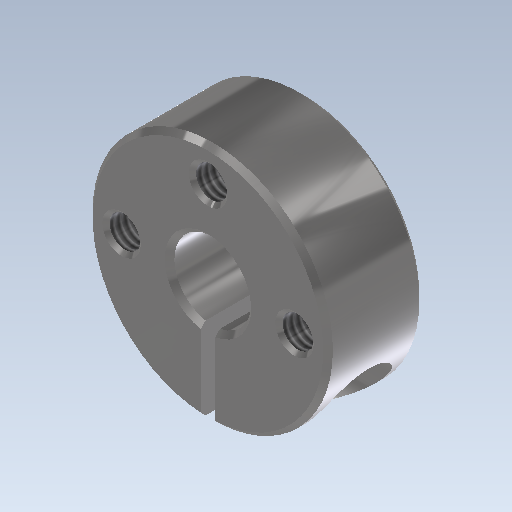
# Autodesk Inventor part: SCSTR8-10b
Saved by Autodesk Inventor 2020 (Build 240168000, 168)
## iProperties
Created: 2019-10-10
Part Number: SCSTR8-10b
Material: 鋼、炭素鋼
Catalog Web Link: www.cadenas.de
Description: SCST, PSCST, SSCST, SCSTR, PSCSTR, SSCSTR-b-Shaft Collars - 3 Holes/3 Taps
Vendor: MISUMI
Document SubType Name: Modeling
Designer: psadmin
Manufacturer: MISUMI
Mass: 28.8211 g
Surface Area: 23.8751 cm^2
Volume: 3.67148 cm^3
Density: 7.85 g/cm^3
Appearance: 半つや出し
Category: PARTsolutions
Company: MISUMI
PSOL_IDENT_0: {$CADENAS_DATA\23d-libs\misumi\metric\03_set_collars\scst\scst_b.prj},210 {VTYP=3D},{NB=SCSTR8-10b},
PSOL_IDENT_1: {LINA=SCSTR8-10},{NN=SCST, PSCST, SSCST, SCSTR, PSCSTR, SSCSTR-b},{DATE=30.03.2018 01:14:48},{GEOMDA
PSOL_IDENT_2: TE=30.10.2015 01:43:51},{VERSION=},{LINEID=50},{WBVAR=TS,MAT,ST,BS},{WBNUMERIC=BS}  {NB=SCSTR8-10b},
PSOL_IDENT_3: {LINA=SCSTR8-10},{KT=DUMMY},{PN=SCSTR8-10},{TYPE=SCSTR},{TS=3T},{TSALG= '3H' , '3-Hole' , '3T' , '3-
PSOL_IDENT_4: Tapped' },{TSA='3H', '3-Hole', '3T', '3 Tap (Coarse)'},{MAT=S45C},{ST=BO},{STALG= 'BO' , 'Black Oxid
PSOL_IDENT_5: e' , 'ENP' , 'Electroless Nickel Plating' },{AC=Hex Socket Head Cap Screw 1 pc.},{ACMAT=4137 Alloy S
PSOL_IDENT_6: teel},{D=8},{BS=10},{BALG= 8 , 10 },{D1=25},{M=M4},{M3D=4},{DD=4.5},{R=3.75},{W=1.5},{X=8.0},{Y=5},{
PSOL_IDENT_7: P=18},{C=0.5},{S=0.0},{M1=M4},{M13D=4},{L=12}
NN: SCST, PSCST, SSCST, SCSTR, PSCSTR, SSCSTR-b
NT: Shaft Collars - 3 Holes/3 Taps
NB: SCSTR8-10b
NBSYN: $PN.b
LINA: SCSTR8-10
PN: SCSTR8-10
TS: 3-Tapped
MAT: 1045 Carbon Steel
ST: Black Oxide
AC: Hex Socket Head Cap Screw 1 pc.
ACMAT: 4137 Alloy Steel
D: 8
BS: 10
D1: 25
M: M4
DD: 4.5
R: 3.75
W: 1.5
X: 8
Y: 5
P: 18
C: 0.5
S: 0
M1: M4
SUPPLIER: MISUMI
ARTICLENO: SCSTR8-10b
BOMINFO: SCSTR8-10
CREATOR: CADENAS GmbH
Title: SCSTR8-10
Author: Cadenas PARTsolutions
Comments: Shaft Collars - 3 Holes/3 Taps
Autodesk Inventor part; units mm, degrees
sketch "Sketch_14" plane through (0, 0, 0) normal (1, 0, 0) x (0, 1, 0)
  line L0 (0, -5) -> (0, 5)
  line L1 (0, 5) -> (12, 5)
  line L2 (12, 5) -> (12.5, 4.5)
  line L3 (12.5, 4.5) -> (12.5, -4.5)
  line L4 (12.5, -4.5) -> (12, -5)
  line L5 (12, -5) -> (0, -5)
  line L6 (0, -5) -> (0, 5)
  constraints: 14 end point
revolve "Revolution1" add sketch "Sketch_14" angle 360 about axis through (0, 0, -5) along (0, 0, -1)
sketch "Sketch_15" plane through (0, 0, 0) normal (1, 0, 0) x (0, 1, 0)
  line L0 (0, -5) -> (0, 5)
  line L1 (0, 5) -> (4.5, 5)
  line L2 (4.5, 5) -> (4, 4.5)
  line L3 (4, 4.5) -> (4, -4.5)
  line L4 (4, -4.5) -> (4.5, -5)
  line L5 (4.5, -5) -> (0, -5)
  line L6 (0, -5) -> (0, 5)
  constraints: 14 end point
revolve "Revolution2" cut sketch "Sketch_15" angle 360 about axis through (0, 0, -5) along (0, 0, -1)
sketch "Sketch_16" plane through (0, 0, 0) normal (0, 0, 1) x (1, 0, 0)
  arc A0 (-0.75, -13.4792) -> (0.75, -13.4792) centre (0, 0) ccw
  line L0 (0.75, -13.4792) -> (0.75, 0)
  line L1 (0.75, 0) -> (-0.75, 0)
  line L2 (-0.75, 0) -> (-0.75, -13.4792)
  constraints: 6 end point, 2 point on circle, 1 centre point
extrude "Extrusion1" cut sketch "Sketch_16" along normal mid plane 10
sketch "Sketch_18" plane through (9, 0, 0) normal (1, 0, 0) x (0, 0, -1)
  line L0 (5, 0) -> (-5, 0)
  line L1 (-5, 0) -> (-5, 2)
  line L2 (-5, 2) -> (-4.621, 1.621)
  line L3 (-4.621, 1.621) -> (4.621, 1.621)
  line L4 (4.621, 1.621) -> (5, 2)
  line L5 (5, 2) -> (5, 0)
  line L6 (5, 0) -> (-5, 0)
  constraints: 14 end point
revolve "Revolution3" cut sketch "Sketch_18" angle 360 about axis through (9, 0, -5) along (0, 0, -1)
thread "Thread1" size "M4x0.7" class "6H" standard "ISO Metric profile" full length
sketch "Sketch_20" plane through (-9, 0, 0) normal (1, 0, 0) x (0, 0, -1)
  line L0 (5, 0) -> (-5, 0)
  line L1 (-5, 0) -> (-5, 2)
  line L2 (-5, 2) -> (-4.621, 1.621)
  line L3 (-4.621, 1.621) -> (4.621, 1.621)
  line L4 (4.621, 1.621) -> (5, 2)
  line L5 (5, 2) -> (5, 0)
  line L6 (5, 0) -> (-5, 0)
  constraints: 14 end point
revolve "Revolution4" cut sketch "Sketch_20" angle 360 about axis through (-9, 0, -5) along (0, 0, -1)
thread "Thread2" size "M4x0.7" class "6H" standard "ISO Metric profile" full length
sketch "Sketch_22" plane through (0, 9, 0) normal (0, 1, 0) x (1, 0, 0)
  line L0 (0, 5) -> (0, -5)
  line L1 (0, -5) -> (-2, -5)
  line L2 (-2, -5) -> (-1.621, -4.621)
  line L3 (-1.621, -4.621) -> (-1.621, 4.621)
  line L4 (-1.621, 4.621) -> (-2, 5)
  line L5 (-2, 5) -> (0, 5)
  line L6 (0, 5) -> (0, -5)
  constraints: 14 end point
revolve "Revolution5" cut sketch "Sketch_22" angle 360 about axis through (0, 9, -5) along (0, 0, -1)
thread "Thread3" size "M4x0.7" class "6H" standard "ISO Metric profile" full length
sketch "Sketch_23" plane through (0, -8, 0) normal (0, 1, 0) x (1, 0, 0)
  line L0 (12.5, 0) -> (0, 0)
  line L1 (0, 0) -> (0, 2.25)
  line L2 (0, 2.25) -> (5, 2.25)
  line L3 (5, 2.25) -> (5, 3.75)
  line L4 (5, 3.75) -> (12.5, 3.75)
  line L5 (12.5, 3.75) -> (12.5, 0)
  line L6 (12.5, 0) -> (0, 0)
  constraints: 14 end point
revolve "Revolution6" cut sketch "Sketch_23" angle 360 about axis through (12.5, -8, 0) along (1, 0, 0)
sketch "Sketch_25" plane through (0, 0, 0) normal (0, 0, 1) x (1, 0, 0)
  line L0 (-0.75, -8) -> (-10.9659, -8)
  line L1 (-10.9659, -8) -> (-10.9659, -6.379)
  line L2 (-10.9659, -6.379) -> (-1.129, -6.379)
  line L3 (-1.129, -6.379) -> (-0.75, -6)
  line L4 (-0.75, -6) -> (-0.75, -8)
  line L5 (-0.75, -8) -> (-10.9659, -8)
  constraints: 12 end point
revolve "Revolution7" cut sketch "Sketch_25" angle 360 about axis through (-0.75, -8, 0) along (1, 0, 0)
thread "Thread4" size "M4x0.7" class "6H" standard "ISO Metric profile" length 9.8369
ref_plane "to_bolt_XY" through (5, -8, 0) normal (1, 0, 0) x (0, 0, -1)
ref_plane "to_bolt_YZ" through (5, -8, 0) normal (0, 0, -1) x (0, 1, 0)
ref_plane "to_bolt_ZX" through (5, -8, 0) normal (0, 1, 0) x (1, 0, 0)
body "Solid1"
